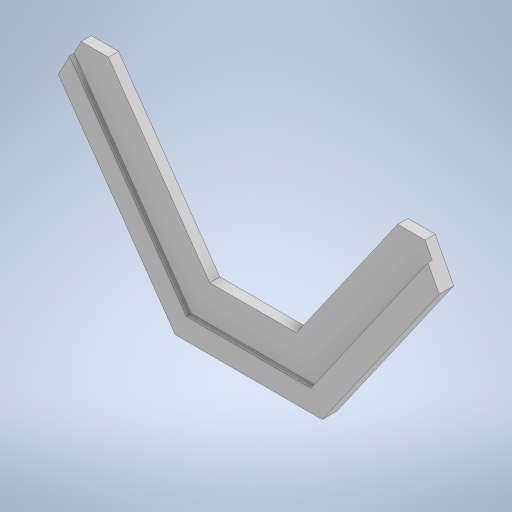
# Autodesk Inventor part: ДМС 045 держатель лотка
Saved by Autodesk Inventor 2024.2 (Build 282272000, 272)
## iProperties
Created: 2024-05-13
Part Number: ДМС 045 держатель лотка
Material: Generic
Document SubType Name: Modeling
Designer: admin
Density: 1 g/cm^3
Appearance: Default
Author: admin
Autodesk Inventor part; units mm, degrees
ref_plane "YZ Plane" through (0, 0, 0) normal (1, 0, 0) x (0, 1, 0)
ref_plane "XZ Plane" through (0, 0, 0) normal (0, 1, 0) x (-1, 0, 0)
ref_plane "XY Plane" through (0, 0, 0) normal (0, 0, 1) x (1, 0, 0)
sketch "Sketch1" plane through (0, 0, 0) normal (0, 1, 0) x (-1, 0, 0)
  line L0 (100, 100) -> (-100, 100) construction
  line L1 (-30, 0) -> (30, 0)
  line L2 (-30, 0) -> (-100, 100)
  line L3 (100, 100) -> (30, 0)
  line L4 (100, 100) -> (148.8262, 100)
  line L5 (148.8262, 100) -> (50.8262, -40)
  line L6 (50.8262, -40) -> (-50.8262, -40)
  line L7 (-50.8262, -40) -> (-148.8262, 100)
  line L8 (-148.8262, 100) -> (-100, 100)
  point P0 (0, 0)
  point P1 (0, 0)
  point P2 (0, 100)
  point P3 (0, -40)
  dimension "d0" = 200
  dimension "d1" = 60
  dimension "d2" = 100
  dimension "d3" = 40
  dimension "d5" = 40
  constraints: 18 end point, 3 horizontal, 3 midpoint, 3 parallel, 2 vertical alignment, 1 coincident, 1 collinear, 1 point on line
  measures "d0" distance of L0.start L0.end
  measures "d1" distance of L1.start L1.end
  measures "d2" distance between parallel lines of L1 L0
  measures "d3" distance between parallel lines of L6 L1
  measures "d5" distance between parallel lines of L5 L3
extrude "Extrusion1" add sketch "Sketch1" along normal blind 10
sketch "Sketch2" plane through (0, 0, 0) normal (0, -1, 0) x (1, 0, 0)
  line L0 (-30, 0) -> (30, 0) projected
  line L1 (-100, 100) -> (-30, 0) projected
  line L2 (-148.8262, 100) -> (-100, 100) projected
  line L3 (-50.8262, -40) -> (-148.8262, 100) construction
  line L4 (50.8262, -40) -> (-50.8262, -40) construction
  line L5 (148.8262, 100) -> (50.8262, -40) construction
  line L6 (100, 100) -> (148.8262, 100) projected
  line L7 (30, 0) -> (100, 100) projected
  line L8 (-130.5164, 100) -> (-43.0164, -25)
  line L9 (-43.0164, -25) -> (43.0164, -25)
  line L10 (43.0164, -25) -> (130.5164, 100)
  line L11 (100, 100) -> (148.8262, 100) projected
  line L12 (-100, 100) -> (-30, 0) projected
  line L13 (30, 0) -> (100, 100) projected
  point P0 (0, 0)
  dimension "d8" = 25
  dimension "d9" = 25
  dimension "d10" = 25
  constraints: 6 end point, 2 parallel, 2 point on line, 1 horizontal
  measures "d8" distance between parallel lines of L9 L0
  measures "d9" distance between parallel lines of L1 L8
  measures "d10" distance between parallel lines of L7 L10
extrude "Extrusion2" cut sketch "Sketch2" against normal blind 3
chamfer "Chamfer1" distance 30 angle 45 2 edges at (148.8262, 5, 100) (-148.8262, 5, 100)
equation "\"d5\" = d3"
equation "\"d9\" = d8"
equation "\"d10\" = d8"
body "Solid1"
